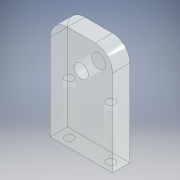
# Autodesk Inventor part: Z-Kettenhalter3
Saved by Autodesk Inventor 2021.3 (Build 253353000, 353)
## iProperties
Created: 2021-04-27
Part Number: Z-Kettenhalter3
Material: Generic
Document SubType Name: Modeling
Designer: Fabijan_Sven
Density: 1 g/cm^3
Appearance: Clear
Author: Fabijan_Sven
Autodesk Inventor part; units mm, degrees
ref_plane "YZ Plane" through (0, 0, 0) normal (1, 0, 0) x (0, 1, 0)
ref_plane "XZ Plane" through (0, 0, 0) normal (0, 1, 0) x (-1, 0, 0)
ref_plane "XY Plane" through (0, 0, 0) normal (0, 0, 1) x (1, 0, 0)
sketch "Sketch1" plane through (0, 0, 0) normal (0, 0, 1) x (1, 0, 0)
  line L0 (0, 0) -> (0, 5) projected
  line L1 (18, 0) -> (18, 5) projected
  line L2 (0, 0) -> (18, 0) projected
  line L3 (0, 0) -> (18, 0)
  line L4 (18, 0) -> (18, 30)
  line L5 (18, 30) -> (0, 30)
  line L6 (0, 30) -> (0, 0)
  dimension "d0" = 30
  constraints: 8 end point, 2 parallel, 1 collinear, 1 horizontal, 1 perpendicular
  measures "d0" distance of L3.end L4.end
extrude "Extrusion1" add sketch "Sketch1" along normal blind 5
fillet "Fillet1" radius 5 2 edges at (0, 30, 2.5) (18, 30, 2.5)
sketch "Sketch3" plane through (0, 0, 5) normal (0, 0, 1) x (1, 0, 0)
  circle A0 centre (9, 21) radius 2
  line L0 (0, 25) -> (0, 0) projected
  line L1 (13, 30) -> (5, 30) projected
  dimension "d11" = 9
  dimension "d12" = 9
  dimension "d13" = 4
  constraints: 1 centre point
  measures "d11" distance from line of L0 A0.centre
  measures "d12" distance from line of A0.centre L1
  measures "d13" diameter of A0
hole "Hole2" at (9, 21, 5) direction (0, 0, -1) diameter 4 depth 20 tip angle 118
sketch "Sketch4" plane through (0, 0, 0) normal (0, -1, 0) x (1, 0, 0)
  circle A0 centre (3, 2.5) radius 1.5
  circle A1 centre (15, 2.5) radius 1.5
  line L0 (0, 0) -> (18, 0) projected
  line L1 (0, 0) -> (0, 5) projected
  dimension "d21" = 12
  dimension "d22" = 2.5
  dimension "d23" = 2.5
  dimension "d24" = 3
  dimension "d25" = 3
  dimension "d26" = 3
  constraints: 2 centre point
  measures "d21" distance of A1.centre A0.centre
  measures "d22" distance from line of L0 A0.centre
  measures "d23" distance from line of L0 A1.centre
  measures "d24" distance from line of L1 A0.centre
  measures "d25" diameter of A0
  measures "d26" diameter of A1
hole "Hole3" at (3, 0, 2.5) at (15, 0, 2.5) direction (0, 1, 0) diameter 2.459 depth 15 tip angle 118 thread size "M3x0.5" class "6H" standard "ISO Metric profile"
equation "\"d14\" = d13"
body "Solid1"
